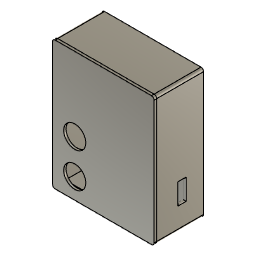
Casing (Autodesk Fusion 360 design; units mm, degrees)
Autodesk Fusion 360 part; units mm, degrees
note: some values were not read from the file. Set by a fixed rule: which face or edge a step refers to.
sketch "Sketch1" plane through (0, 0, 0) normal (0, 0, 1) x (1, 0, 0) in component "main_body"
  line L0 (0, 0) -> (78, 0)
  line L1 (78, 0) -> (78, 59)
  line L2 (78, 59) -> (0, 59)
  line L3 (0, 59) -> (0, 0)
  dimension "d5" = 78
  dimension "d6" = 59
  constraint horizontal L0
  constraint vertical L1
  constraint horizontal L2
  constraint vertical L3
  constraint coincident L0.start L3.end
  measures "d5" distance of L0.start L0.end
  measures "d6" distance of L0.start L2.end
extrude "Extrude1" add sketch "Sketch1" along normal blind 99 makes body 1 in component "main_body"
shell "Shell1" thickness 2 removed faces 1 at (26, 0, 33) on bodies 1 in component "main_body"
extrude "Extrude2" cut 1 faces at (51.3333, 57, 65.3333) along direction (0, 1, 0) blind 215 on bodies 1 bodies 1 in component "main_body"
sketch "Sketch2" plane through (0, 0, 2) normal (0, 0, 1) x (-1, 0, 0) in component "main_body"
  line L0 (-2, -59) -> (-2, 0)
  line L1 (-76, 0) -> (-76, -59)
  line L2 (-76, -59) -> (-2, -59)
  line L3 (-2, -59) -> (-2, -58)
  line L4 (-2, -59) -> (-2, -37)
  line L5 (-2, -37) -> (-76, -37)
  line L6 (-76, -37) -> (-76, -35)
  line L7 (-76, -35) -> (-2, -35)
  dimension "d12" = 22
  dimension "d13" = 2
  constraint coincident L0.start L2.end
  constraint coincident L0 L3.end
  constraint perpendicular L2 L3
  constraint perpendicular L2 L4
  constraint horizontal L5
  constraint coincident L1 L5.end
  constraint coincident L1 L6.end
  constraint coincident L0 L7.end
  constraint perpendicular L0 L7
  measures "d12" distance of L0.start L4.end
  measures "d13" distance of L5.end L6.end
extrude "Extrude3" cut 1 faces at (0.6667, 0, 33.6667) along direction (0, 1, 0) blind 8 on bodies 1 bodies 1 in component "main_body"
extrude "Extrude4" add sketch "Sketch2" along normal blind 55.2 contours L0 L1 L5 L6 L7 bodies 1 in component "main_body"
extrude "Extrude5" add 1 faces at (0.6667, 8, 33.6667) along direction (0, -1, 0) blind 1 on bodies 1 bodies 1 in component "main_body"
extrude "Extrude6" add 1 faces at (0.6667, 7, 33.6667) along direction (0, -1, 0) blind 0.5 on bodies 1 bodies 1 in component "main_body"
sketch "Sketch3" plane through (0, 35, 0) normal (0, -1, 0) x (1, 0, 0) in component "main_body"
  line L0 (2, 57.2) -> (2, 2)
  line L1 (2, 2) -> (76, 2)
  line L2 (76, 2) -> (76, 57.2)
  line L3 (2, 57.2) -> (7, 57.2)
  line L4 (7, 57.2) -> (7, 2)
  line L5 (7, 2) -> (2, 2)
  line L6 (2, 2) -> (2, 57.2)
  line L7 (7, 2) -> (76, 2)
  line L8 (76, 2) -> (76, 5)
  line L9 (76, 5) -> (7, 5)
  line L10 (7, 5) -> (7, 2)
  line L11 (7, 57.2) -> (76, 57.2)
  line L12 (76, 57.2) -> (76, 53.2)
  line L13 (76, 53.2) -> (7, 53.2)
  line L14 (7, 53.2) -> (7, 57.2)
  line L15 (7, 53.2) -> (27.2, 53.2)
  line L16 (27.2, 53.2) -> (27.2, 5)
  line L17 (27.2, 5) -> (7, 5)
  line L18 (7, 5) -> (7, 53.2)
  line L19 (9, 51.2) -> (25.2, 51.2)
  line L20 (25.2, 51.2) -> (25.2, 7)
  line L21 (25.2, 7) -> (9, 7)
  line L22 (9, 7) -> (9, 51.2)
  circle A0 centre (17.1, 42.3) radius 8.1
  circle A1 centre (17.1, 15.7) radius 8.1
  line L23 (76, 5) -> (76, 11.4)
  line L24 (76, 53.2) -> (76, 39.8)
  line L25 (76, 39.8) -> (76, 32.8)
  line L26 (76, 11.4) -> (76, 18.4)
  line L27 (76, 57.2) -> (76, 2)
  line L28 (76, 2) -> (76, 97)
  line L29 (2, 57.2) -> (6, 57.2)
  line L30 (6, 57.2) -> (6, 53.2)
  line L31 (6, 53.2) -> (2, 53.2)
  line L32 (2, 53.2) -> (2, 57.2)
  line L33 (76, 57.2) -> (2, 57.2)
  line L34 (76, 2) -> (76, 57.2)
  line L35 (76, 97) -> (76, 2)
  dimension "d22" = 5
  dimension "d23" = 3
  dimension "d24" = 4
  dimension "d27" = 20.2
  dimension "d28" = 2
  dimension "d29" = 16.2
  dimension "d30" = 16.2
  dimension "d31" = 6.4
  dimension "d32" = 13.4
  dimension "d33" = 7
  dimension "d34" = 7
  dimension "d97" = 4
  dimension "d98" = 4
  constraint horizontal L3
  constraint vertical L4
  constraint horizontal L5
  constraint vertical L6
  constraint coincident L1 L4.end
  constraint coincident L0.start L3.start
  constraint horizontal L7
  constraint vertical L8
  constraint horizontal L9
  constraint vertical L10
  constraint coincident L2 L8.end
  constraint horizontal L11
  constraint vertical L12
  constraint horizontal L13
  constraint vertical L14
  constraint coincident L2 L12.end
  constraint horizontal L15
  constraint vertical L16
  constraint horizontal L17
  constraint vertical L18
  constraint coincident L9 L16.end
  constraint perpendicular L9 L23
  constraint perpendicular L13 L24
  constraint perpendicular L11 L25
  constraint parallel L2 L26
  constraint horizontal L29
  constraint vertical L30
  constraint horizontal L31
  constraint vertical L32
  measures "d22" distance of L0.start L3.end
  measures "d23" distance of L4.end L9.end
  measures "d24" distance of L3.end L13.end
  measures "d27" distance of L13.end L15.end
  measures "d29" diameter of A0
  measures "d30" diameter of A1
  measures "d31" distance of L8.end L23.end
  measures "d32" distance of L12.end L24.end
  measures "d33" distance of L24.end L25.end
  measures "d34" distance of L23.end L26.end
  measures "d97" distance of L0.start L29.end
  measures "d98" distance of L0.start L31.end
extrude "Extrude7" add 1 faces at (0.6667, 6.5, 33.6667) along direction (0, -1, 0) blind 1.5 on bodies 1 bodies 1 in component "main_body"
sketch "Sketch4" plane through (76, 0, 0) normal (-1, 0, 0) x (0, -1, 0) in component "main_body"
  line L0 (-35, 57.2) -> (-35, 2)
  line L1 (-35, 2) -> (-5, 2)
  line L2 (-5, 2) -> (-5, 97)
  line L3 (-5, 97) -> (-59, 97)
  line L4 (-37, 2) -> (-37, 57.2)
  line L5 (-37, 57.2) -> (-35, 57.2)
  line L6 (-59, 97) -> (-59, 2)
  line L7 (-59, 2) -> (-37, 2)
sketch "Sketch5" plane through (76, 0, 0) normal (-1, 0, 0) x (0, -1, 0) in component "main_body"
  line L0 (-35, 18.4) -> (-35, 32.6)
  line L1 (-35, 32.6) -> (-21.7, 32.6)
  line L2 (-21.7, 32.6) -> (-22.7, 32.6)
  line L3 (-35, 18.4) -> (-22.7, 18.4)
  line L4 (-22.7, 18.4) -> (-22.7, 32.6)
  line L5 (-22.7, 32.6) -> (-35, 32.6)
  line L6 (-35, 32.6) -> (-35, 18.4)
  line L7 (-22.7, 32.6) -> (-18.2, 32.6)
  line L8 (-18.2, 32.6) -> (-18.2, 18.4)
  line L9 (-18.2, 18.4) -> (-22.7, 18.4)
  line L10 (-22.7, 18.4) -> (-22.7, 32.6)
  dimension "d36" = 13.3
  dimension "d37" = 1
  dimension "d38" = 4.5
  constraint vertical L0
  constraint perpendicular L0 L2
  constraint horizontal L3
  constraint vertical L4
  constraint horizontal L5
  constraint vertical L6
  constraint horizontal L7
  constraint vertical L8
  constraint horizontal L9
  constraint vertical L10
  measures "d36" distance of L0.end L1.end
  measures "d37" distance of L1.end L2.end
  measures "d38" distance of L2.end L7.end
extrude "Extrude8" cut sketch "Sketch5" against normal blind 13 contours L1 L2 L4 L7 L8 L9 L10 bodies 1 in component "main_body"
fillet "Fillet1" radius 1 8 edges at (76, 22.7, 25.5) (76, 20.45, 18.4) (78, 22.7, 25.5) (76, 20.45, 32.6) (76, 18.2, 25.5) (78, 20.45, 32.6) (78, 18.2, 25.5) (78, 20.45, 18.4) on bodies 1 in component "main_body"
extrude "Extrude9" add 1 faces at (0.6667, 5, 33.6667) along direction (0, -1, 0) blind 3 on bodies 1 bodies 1 in component "main_body"
extrude "Extrude10" add 1 faces at (0.6667, 2, 33.6667) along direction (0, -1, 0) blind 1 on bodies 1 bodies 1 in component "main_body"
sketch "Sketch7" plane through (0, 0, 2) normal (0, 0, 1) x (-1, 0, 0) in component "main_body"
  line L0 (-76, -35) -> (-2, -35)
  line L1 (-2, -35) -> (-2, -1)
  line L2 (-2, -1) -> (-76, -1)
  line L3 (-76, -1) -> (-76, -35)
  line L4 (-39, -1) -> (-24, -1)
  line L5 (-24, -1) -> (-24, -4.5)
  line L6 (-24, -4.5) -> (-39, -4.5)
  line L7 (-39, -4.5) -> (-39, -1)
  line L8 (-39, -1) -> (-54, -1)
  line L9 (-54, -1) -> (-54, -4.5)
  line L10 (-54, -4.5) -> (-39, -4.5)
  line L11 (-39, -4.5) -> (-39, -1)
  dimension "d47" = 15
  dimension "d48" = 3.5
  dimension "d49" = 3.5
  constraint horizontal L4
  constraint vertical L5
  constraint horizontal L6
  constraint vertical L7
  constraint midpoint L2 L4.start
  constraint horizontal L8
  constraint vertical L9
  constraint horizontal L10
  constraint vertical L11
  measures "d47" distance of L4.start L4.end
  measures "d48" distance of L4.start L6.end
  measures "d49" distance of L4.start L6.end
extrude "Extrude11" add sketch "Sketch7" along normal blind 7 draft -45 contours L2 L7 L8 L9 L10 L11 | L2 L4 L5 L6 L7 L11 bodies 1 in component "main_body"
ref_plane "WorkPlane1" through (39, 18, 49.5) normal (0, 0, 1) x (1, 0, 0) in component "main_body"
mirror "Mirror1" about plane through (39, 18, 49.5) normal (0, 0, 1) of "Extrude11" in component "main_body"
fillet "Fillet2" radius 2 4 edges at (0, 30, 99) (78, 30, 99) (78, 30, 0) (0, 30, 0) on bodies 1 in component "main_body"
sketch "Sketch2 (2)" plane through (0, 0.5264, 0) normal (0, -1, 0) x (1, 0, 0) in component "front_closure"
  line L0 (1.4681, 1.8275) -> (1.4681, 96.8275)
  line L1 (1.4681, 96.8275) -> (23.4681, 96.8275)
  line L2 (23.4681, 96.8275) -> (53.4681, 96.8275)
  line L3 (53.4681, 96.8275) -> (75.4681, 96.8275)
  line L4 (75.4681, 96.8275) -> (75.4681, 1.8275)
  line L5 (75.4681, 1.8275) -> (53.4681, 1.8275)
  line L6 (53.4681, 1.8275) -> (23.4681, 1.8275)
  line L7 (23.4681, 1.8275) -> (1.4681, 1.8275)
  arc A0 (-0.5319, 1.8275) -> (1.4681, -0.1725) centre (1.4681, 1.8275) ccw
  line L8 (1.4681, -0.1725) -> (75.4681, -0.1725)
  arc A1 (75.4681, -0.1725) -> (77.4681, 1.8275) centre (75.4681, 1.8275) ccw
  line L9 (77.4681, 1.8275) -> (77.4681, 96.8275)
  arc A2 (77.4681, 96.8275) -> (75.4681, 98.8275) centre (75.4681, 96.8275) ccw
  line L10 (75.4681, 98.8275) -> (1.4681, 98.8275)
  arc A3 (1.4681, 98.8275) -> (-0.5319, 96.8275) centre (1.4681, 96.8275) ccw
  line L11 (-0.5319, 96.8275) -> (-0.5319, 1.8275)
extrude "Extrude2'" add sketch "Sketch2 (2)" along normal blind 2 separate body contours L0 L1 L2 L3 L4 L5 L6 L7 | A0 L8 A1 L9 A2 L10 A3 L11 makes body 2 in component "front_closure"
sketch "Sketch3 (2)" plane through (0, 0.5264, 0) normal (0, 1, 0) x (-1, 0, 0) in component "front_closure"
  line L0 (0.5319, 1.8275) -> (0.5319, 96.8275)
  arc A0 (0.5319, 96.8275) -> (-1.4681, 98.8275) centre (-1.4681, 96.8275) ccw
  line L1 (-1.4681, 98.8275) -> (-75.4681, 98.8275)
  arc A1 (-75.4681, 98.8275) -> (-77.4681, 96.8275) centre (-75.4681, 96.8275) ccw
  line L2 (-77.4681, 96.8275) -> (-77.4681, 1.8275)
  arc A2 (-77.4681, 1.8275) -> (-75.4681, -0.1725) centre (-75.4681, 1.8275) ccw
  line L3 (-75.4681, -0.1725) -> (-1.4681, -0.1725)
  arc A3 (-1.4681, -0.1725) -> (0.5319, 1.8275) centre (-1.4681, 1.8275) ccw
  line L4 (-75.1681, 96.5275) -> (-75.1681, 2.1275)
  line L5 (-75.1681, 2.1275) -> (-1.7681, 2.1275)
  line L6 (-1.7681, 2.1275) -> (-1.7681, 96.5275)
  line L7 (-1.7681, 96.5275) -> (-75.1681, 96.5275)
extrude "Extrude3'" add sketch "Sketch3 (2)" along normal blind 4 contours L4 L5 L6 L7 bodies 2 in component "front_closure"
extrude "Extrude4'" cut 1 faces at (50.7014, 4.5264, 33.5941) along direction (0, -1, 0) blind 0.5 on bodies 2 bodies 2 in component "front_closure"
extrude "Extrude5'" cut sketch "Sketch7" along normal blind 2.5 draft -45 from surface at 0.3 contours L2 L7 L8 L9 L10 L11 | L2 L4 L5 L6 L7 L11 sketch seen with x (1, 0, 0) y (0, 1, 0) z (0, 0, 1) at (-0.5319, -0.4736, -0.1725) bodies 2 in component "front_closure"
mirror "Mirror1'" about plane through (38.4681, 17.5264, 49.3275) normal (0, 0, 1) of "Extrude5'" in component "front_closure"
shell "Shell1'" thickness 2 removed faces 1 at (43.4681, 4.0264, 33.5941) on bodies 2 in component "front_closure"
chamfer "Chamfer1" distance 0.6 angle 45 1 edges at (38.4681, 4.0264, 96.5275) on bodies 2 in component "front_closure"
chamfer "Chamfer2" distance 0.6 angle 45 1 edges at (38.4681, 4.0264, 2.1275) on bodies 2 in component "front_closure"
fillet "Fillet1'" radius 1 4 edges at (1.7681, 2.2764, 96.5275) (1.7681, 2.2764, 2.1275) (75.1681, 2.2764, 96.5275) (75.1681, 2.2764, 2.1275) on bodies 2 in component "front_closure"
sketch "Sketch9" plane through (0, 37, 0) normal (0, 1, 0) x (-1, 0, 0) in component "main_body"
  line L0 (-76, 57.2) -> (-76, 2)
  line L1 (-76, 2) -> (-2, 2)
  line L2 (-2, 2) -> (-2, 57.2)
  line L3 (-2, 57.2) -> (-6, 57.2)
  line L4 (-6, 57.2) -> (-6, 53.2)
  line L5 (-6, 53.2) -> (-2, 53.2)
  line L6 (-2, 53.2) -> (-2, 57.2)
  line L7 (-2, 57.2) -> (-76, 57.2)
  dimension "d101" = 4
  dimension "d102" = 4
  constraint horizontal L3
  constraint vertical L4
  constraint horizontal L5
  constraint vertical L6
  constraint coincident L2.end L3.start
  measures "d101" distance of L2.end L3.end
  measures "d102" distance of L2.end L5.end
extrude "Extrude14" cut sketch "Sketch9" against normal blind 20 contours L2 L3 L4 L5 L6 L7 bodies 1 in component "main_body"
extrude "Extrude7'" cut sketch "Sketch3" along normal blind 85 contours A0 | A1 sketch seen with x (1, 0, 0) y (0, 1, 0) z (0, 0, 1) at (-0.5319, -0.4736, -0.1725) bodies 2 in component "front_closure"
fillet "Fillet2'" radius 1 2 edges at (9.0163, 0.5264, 39.1984) (9.0163, 0.5264, 12.5984) on bodies 2 in component "front_closure"
extrude "Extrude15" add 1 faces at (0.6667, 59, 65.3333) along direction (0, 1, 0) blind 3.5 on bodies 1 bodies 1 in component "main_body"
sketch "Sketch1 (2)" plane through (0, 0, 1.8275) normal (0, 0, 1) x (-1, 0, 0)
  line L0 (-1.4681, -36.5264) -> (-75.4681, -36.5264)
  line L1 (-75.4681, -36.5264) -> (-75.4681, -62.0264)
  line L2 (-75.4681, -62.0264) -> (-1.4681, -62.0264)
  line L3 (-1.4681, -62.0264) -> (-1.4681, -36.5264)
  line L4 (-38.4681, -62.0264) -> (-53.4681, -62.0264)
  line L5 (-53.4681, -62.0264) -> (-53.4681, -58.5264)
  line L6 (-53.4681, -58.5264) -> (-38.4681, -58.5264)
  line L7 (-38.4681, -58.5264) -> (-38.4681, -62.0264)
  line L8 (-38.4681, -62.0264) -> (-23.4681, -62.0264)
  line L9 (-23.4681, -62.0264) -> (-23.4681, -58.5264)
  line L10 (-23.4681, -58.5264) -> (-38.4681, -58.5264)
  line L11 (-38.4681, -58.5264) -> (-38.4681, -62.0264)
  dimension "d113" = 15
  dimension "d114" = 3.5
  dimension "d115" = 3.5
  constraint horizontal L4
  constraint vertical L5
  constraint horizontal L6
  constraint vertical L7
  constraint midpoint L2 L4.start
  constraint horizontal L8
  constraint vertical L9
  constraint horizontal L10
  constraint vertical L11
  measures "d113" distance of L4.start L4.end
  measures "d114" distance of L4.start L6.end
  measures "d115" distance of L4.start L6.end
extrude "Extrude17" add 1 faces at (4.6667, 36.3333, 53.2) along direction (0, 0, 1) blind 4 on bodies 1 bodies 1 in component "main_body"
extrude "Extrude18" add 1 faces at (26.6667, 35.6667, 57.2) along direction (0, 0, 1) blind 40 on bodies 1 bodies 1 in component "main_body"
extrude "Extrude20" cut 1 faces at (0.6667, 62.5, 65.3333) along direction (0, -1, 0) blind 25.5 on bodies 1 bodies 1 in component "main_body"
sketch "Sketch2 (3)" plane through (0, -1.4736, 0) normal (0, -1, 0) x (1, 0, 0)
  circle A0 centre (16.5681, 42.1275) radius 8.1
  circle A1 centre (16.5681, 15.5275) radius 8.1
  line L0 (-0.5319, 96.8275) -> (-0.5319, 1.8275)
  arc A2 (-0.5319, 1.8275) -> (1.4681, -0.1725) centre (1.4681, 1.8275) ccw
  line L1 (1.4681, -0.1725) -> (75.4681, -0.1725)
  arc A3 (75.4681, -0.1725) -> (77.4681, 1.8275) centre (75.4681, 1.8275) ccw
  line L2 (77.4681, 1.8275) -> (77.4681, 96.8275)
  arc A4 (77.4681, 96.8275) -> (75.4681, 98.8275) centre (75.4681, 96.8275) ccw
  line L3 (75.4681, 98.8275) -> (1.4681, 98.8275)
  arc A5 (1.4681, 98.8275) -> (-0.5319, 96.8275) centre (1.4681, 96.8275) ccw
  circle A6 centre (16.5681, 15.5275) radius 8.5
  circle A7 centre (16.5681, 42.1275) radius 8.5
  dimension "d142" = 0.4
  dimension "d143" = 0.4
extrude "Extrude8'" cut sketch "Sketch2 (3)" against normal blind 4 contours A6 | A7 bodies 2 in component "front_closure"
extrude "Extrude6'" [suppressed] in component "front_closure"
extrude "Extrude13" [suppressed] in component "main_body"
component "main_body" placed x (1, 0, 0) y (0, 1, 0) z (0, 0, 1) at (-0.5319, -0.4736, -0.1725)
component "front_closure" placed x (1, 0, 0) y (0, 1, 0) z (0, 0, 1) at (0, 0, 0)
equation "width = 55 mm"
equation "length = 74 mm"
equation "shell = 2 mm"
equation "height = 95 mm"
equation "d5 = length + shell * 2"
equation "d6 = width + shell * 2"
equation "d7 = height + shell * 2"
equation "d9 = shell"
equation "d13 = shell"
equation "d58 = shell"
equation "d60 = -( shell + gap )"
equation "gap = 0.3 mm"
equation "d62 = shell * 2"
equation "d88 = shell"
